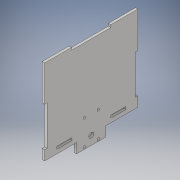
# Autodesk Inventor part: side
Saved by Autodesk Inventor 2019 (Build 230136000, 136)
## iProperties
Created: 2018-09-07
Part Number: side
Material: Generic
Document SubType Name: Modeling
Designer: mspet
Density: 1 g/cm^3
Appearance: Default
Author: mspet
Autodesk Inventor part; units mm, degrees
ref_plane "YZ Plane" through (0, 0, 0) normal (1, 0, 0) x (0, 1, 0)
ref_plane "XZ Plane" through (0, 0, 0) normal (0, 1, 0) x (-1, 0, 0)
ref_plane "XY Plane" through (0, 0, 0) normal (0, 0, 1) x (1, 0, 0)
sketch "Sketch1" plane through (0, 0, 0) normal (1, 0, 0) x (0, 1, 0)
  line L0 (0, 0) -> (97.4344, 0)
  line L1 (97.4344, 0) -> (97.4344, -114.3)
  line L2 (97.4344, -114.3) -> (0, -114.3)
  line L3 (0, -114.3) -> (0, 0)
  dimension "d0" = 114.3
  dimension "d1" = 97.4344
  constraints: 8 end point, 2 parallel, 1 horizontal, 1 perpendicular
  measures "d0" distance of L2.end L0.start
  measures "d1" distance of L1.end L2.end
extrude "Extrusion1" add sketch "Sketch1" along normal blind 3.175
sketch "Sketch2" plane through (3.175, 0, 0) normal (1, 0, 0) x (0, 0, -1)
  circle A0 centre (48.1457, 35.5346) radius 1.4986
  circle A1 centre (66.1543, 35.5346) radius 1.4986
  circle A2 centre (66.1543, 2.54) radius 1.4986
  circle A3 centre (48.1457, 2.54) radius 1.4986
  line L0 (114.3, 0) -> (114.3, 97.4344) projected
  line L1 (0, 0) -> (114.3, 0) projected
  line L2 (0, 0) -> (0, 97.4344) projected
  dimension "d4" = 18.0086
  dimension "d5" = 2.9972
  dimension "d6" = 2.9972
  dimension "d7" = 2.9972
  dimension "d8" = 2.9972
  dimension "d11" = 18.0086
  dimension "d12" = 2.54
  dimension "d28" = 2.54
  dimension "d29" = 32.9946
  dimension "d30" = 32.9946
  dimension "d65" = 48.1457
  constraints: 4 centre point
  measures "d4" distance of A1.centre A0.centre
  measures "d5" diameter of A1
  measures "d6" diameter of A0
  measures "d7" diameter of A3
  measures "d8" diameter of A2
  measures "d11" distance of A2.centre A3.centre
  measures "d12" distance from line of L1 A3.centre
  measures "d28" distance from line of L1 A2.centre
  measures "d29" distance of A2.centre A1.centre
  measures "d30" distance of A3.centre A0.centre
  measures "d65" distance from line of L0 A1.centre
extrude "Extrusion2" cut sketch "Sketch2" against normal blind 3.175
sketch "Sketch3" plane through (3.175, 0, 0) normal (1, 0, 0) x (0, 0, -1)
  circle A0 centre (57.15, 11.5316) radius 3.175
  line L0 (114.3, 0) -> (114.3, 97.4344) projected
  circle A1 centre (66.1543, 2.54) radius 1.4986 projected
  point P0 (0, 0)
  dimension "d15" = 6.35
  dimension "d16" = 57.15
  dimension "d17" = 8.9916
  constraints: 1 centre point
  measures "d15" diameter of A0
  measures "d16" distance from line of L0 A0.centre
  measures "d17" vertical distance of A1.centre A0.centre
extrude "Extrusion3" cut sketch "Sketch3" against normal blind 3.175 contours A0
sketch "Sketch4" plane through (3.175, 0, 0) normal (1, 0, 0) x (0, 0, -1)
  line L0 (0, 97.4344) -> (0, 0) projected
  line L1 (0, 0) -> (114.3, 0) projected
  line L2 (114.3, 0) -> (114.3, 97.4344) projected
  line L3 (31.75, 18.0594) -> (12.7, 18.0594)
  line L4 (12.7, 18.0594) -> (12.7, 21.2344)
  line L5 (12.7, 21.2344) -> (31.75, 21.2344)
  line L6 (31.75, 21.2344) -> (31.75, 18.0594)
  circle A0 centre (57.15, 11.5316) radius 3.175 projected
  line L7 (57.15, 11.5316) -> (57.15, 79.1299) construction
  line L8 (82.55, 18.0594) -> (101.6, 18.0594)
  line L9 (101.6, 18.0594) -> (101.6, 21.2344)
  line L10 (101.6, 21.2344) -> (82.55, 21.2344)
  line L11 (82.55, 21.2344) -> (82.55, 18.0594)
  point P0 (12.7, 0)
  point P1 (31.75, 0)
  point P2 (101.6, 0)
  dimension "d31" = 3.175
  dimension "d33" = 19.05
  dimension "d34" = 12.7
  dimension "d43" = 18.0594
  constraints: 18 end point, 4 symmetric about line, 2 parallel, 1 horizontal, 1 perpendicular, 1 point on line, 1 vertical
  measures "d31" distance of L3.end L4.end
  measures "d33" distance of L4.end L5.end
  measures "d34" distance between parallel lines of L0 L4
  measures "d43" distance between parallel lines of L1 L3
extrude "Extrusion5" cut sketch "Sketch4" against normal blind 3.175 contours L3 L4 L5 L6 | L11 L10 L9 L8
sketch "Sketch5" plane through (3.175, 0, 0) normal (1, 0, 0) x (0, 0, -1)
  line L0 (0, 0) -> (38.1, 0)
  line L1 (38.1, 0) -> (38.1, 12.7)
  line L2 (38.1, 12.7) -> (0, 12.7)
  line L3 (0, 12.7) -> (0, 0)
  line L4 (114.3, 0) -> (0, 0) projected
  line L5 (114.3, 0) -> (76.2, 0)
  line L6 (76.2, 0) -> (76.2, 12.7)
  line L7 (76.2, 12.7) -> (114.3, 12.7)
  line L8 (114.3, 12.7) -> (114.3, 0)
  dimension "d37" = 38.1
  dimension "d38" = 12.7
  dimension "d39" = 38.1
  dimension "d42" = 12.7
  constraints: 16 end point, 4 parallel, 2 horizontal, 2 perpendicular
  measures "d37" distance of L1.end L2.end
  measures "d38" distance of L0.end L1.end
  measures "d39" distance of L6.end L7.end
  measures "d42" distance of L5.end L6.end
extrude "Extrusion6" cut sketch "Sketch5" against normal blind 3.175
sketch "Sketch6" plane through (3.175, 0, 0) normal (1, 0, 0) x (0, 0, -1)
  line L0 (0, 97.4344) -> (0, 12.7) projected
  line L1 (0, 69.85) -> (3.175, 69.85)
  line L2 (3.175, 69.85) -> (3.175, 50.8)
  line L3 (3.175, 50.8) -> (0, 50.8)
  line L4 (0, 50.8) -> (0, 69.85)
  line L5 (0, 12.7) -> (38.1, 12.7) projected
  line L6 (38.1, 0) -> (76.2, 0) projected
  line L7 (57.15, 0) -> (57.15, 76.8026) construction
  line L8 (114.3, 97.4344) -> (114.3, 12.7)
  line L9 (114.3, 69.85) -> (111.125, 69.85)
  line L10 (111.125, 69.85) -> (111.125, 50.8)
  line L11 (111.125, 50.8) -> (114.3, 50.8)
  line L12 (114.3, 50.8) -> (114.3, 69.85)
  point P0 (0, 0)
  dimension "d44" = 38.1
  dimension "d45" = 19.05
  dimension "d46" = 3.175
  constraints: 20 end point, 6 symmetric about line, 2 parallel, 2 point on line, 1 horizontal, 1 midpoint, 1 perpendicular, 1 vertical
  measures "d44" distance between parallel lines of L3 L5
  measures "d45" distance of L1.end L2.end
  measures "d46" distance of L1.start L1.end
extrude "Extrusion7" cut sketch "Sketch6" against normal blind 3.175
sketch "Sketch7" plane through (3.175, 0, 0) normal (1, 0, 0) x (0, 0, -1)
  line L0 (0, 101.4731) -> (-3.175, 101.4731)
  line L1 (-3.175, 101.4731) -> (-3.175, 12.7)
  line L2 (-3.175, 12.7) -> (0, 12.7)
  line L3 (0, 12.7) -> (0, 101.4731)
  line L4 (114.3, 50.8) -> (114.3, 12.7) projected
  line L5 (114.3, 12.7) -> (117.475, 12.7)
  line L6 (117.475, 12.7) -> (117.475, 101.4731)
  line L7 (117.475, 101.4731) -> (114.3, 101.4731)
  line L8 (114.3, 101.4731) -> (114.3, 12.7)
  line L9 (0, 97.4344) -> (0, 69.85) projected
  line L10 (0, 69.85) -> (3.3446, 69.85)
  line L11 (3.3446, 69.85) -> (3.3446, 50.8)
  line L12 (3.3446, 50.8) -> (0, 50.8)
  line L13 (0, 50.8) -> (0, 69.85)
  line L14 (111.125, 69.85) -> (111.125, 50.8) projected
  line L15 (111.125, 69.85) -> (114.3, 69.85)
  line L16 (114.3, 69.85) -> (114.3, 50.8)
  line L17 (114.3, 50.8) -> (111.125, 50.8)
  line L18 (111.125, 50.8) -> (111.125, 69.85)
  line L19 (0, 97.4344) -> (-3.175, 97.4344)
  line L20 (0, 97.4344) -> (114.3, 97.4344) projected
  line L21 (114.3, 97.4344) -> (117.475, 97.4344)
  point P0 (0, 0)
  dimension "d49" = 3.175
  dimension "d50" = 3.175
  dimension "d51" = 0
  constraints: 36 end point, 8 parallel, 6 perpendicular, 4 horizontal, 3 point on line
  measures "d49" distance of L0.start L0.end
  measures "d50" distance of L6.end L7.end
  measures "d51" distance between parallel lines of L9 L3
extrude "Extrusion8" add sketch "Sketch7" against normal blind 3.175
sketch "Sketch8" plane through (3.175, 0, 0) normal (1, 0, 0) x (0, 0, -1)
  line L0 (-3.175, 101.4731) -> (-3.175, 12.7) projected
  line L1 (-3.175, 76.2) -> (0, 76.2)
  line L2 (0, 76.2) -> (0, 25.4)
  line L3 (0, 25.4) -> (-3.175, 25.4)
  line L4 (-3.175, 25.4) -> (-3.175, 76.2)
  line L5 (117.475, 101.4731) -> (117.475, 12.7) projected
  line L6 (117.475, 76.2) -> (114.3, 76.2)
  line L7 (114.3, 76.2) -> (114.3, 25.4)
  line L8 (114.3, 25.4) -> (117.475, 25.4)
  line L9 (117.475, 25.4) -> (117.475, 76.2)
  line L10 (-3.175, 12.7) -> (38.1, 12.7) projected
  point P0 (0, 0)
  dimension "d54" = 3.175
  dimension "d55" = 3.175
  dimension "d56" = 50.8
  dimension "d57" = 50.8
  dimension "d58" = 12.7
  constraints: 16 end point, 4 parallel, 3 point on line, 2 horizontal, 2 perpendicular
  measures "d54" distance of L7.end L8.end
  measures "d55" distance of L1.start L1.end
  measures "d56" distance of L1.end L2.end
  measures "d57" distance of L6.end L7.end
  measures "d58" distance between parallel lines of L10 L3
extrude "Extrusion9" cut sketch "Sketch8" against normal blind 3.175
sketch "Sketch9" plane through (3.175, 0, 0) normal (1, 0, 0) x (0, 0, -1)
  line L0 (-3.175, 76.2) -> (-3.175, 101.4731) projected
  line L1 (-3.175, 97.0871) -> (127.7131, 97.0871)
  line L2 (127.7131, 97.0871) -> (127.7131, 110.1997)
  line L3 (127.7131, 110.1997) -> (-3.175, 110.1997)
  line L4 (-3.175, 110.1997) -> (-3.175, 97.0871)
  point P0 (0, 0)
  constraints: 8 end point, 2 parallel, 1 horizontal, 1 perpendicular, 1 point on line
extrude "Extrusion10" cut sketch "Sketch9" against normal blind 3.175
sketch "Sketch10" plane through (0, 0, 0) normal (-1, 0, 0) x (0, 0, 1)
  line L0 (-117.475, 97.0871) -> (-117.475, 76.2) projected
  line L1 (-117.475, 97.0871) -> (3.175, 97.0871)
  line L2 (3.175, 97.0871) -> (3.175, 122.4871)
  line L3 (3.175, 122.4871) -> (-117.475, 122.4871)
  line L4 (-117.475, 122.4871) -> (-117.475, 97.0871)
  line L5 (3.175, 76.2) -> (3.175, 97.0871) projected
  point P0 (0, 0)
  dimension "d66" = 0
  dimension "d67" = 25.4
  constraints: 8 end point, 2 parallel, 1 horizontal, 1 perpendicular
  measures "d66" distance between parallel lines of L2 L5
  measures "d67" distance of L3.end L0.start
extrude "Extrusion11" add sketch "Sketch10" against normal blind 3.175
sketch "Sketch11" plane through (3.175, 0, 0) normal (1, 0, 0) x (0, 0, -1)
  line L0 (117.475, 122.4871) -> (-3.175, 122.4871) projected
  line L1 (31.75, 122.4871) -> (82.55, 122.4871)
  line L2 (82.55, 122.4871) -> (82.55, 119.3121)
  line L3 (82.55, 119.3121) -> (31.75, 119.3121)
  line L4 (31.75, 119.3121) -> (31.75, 122.4871)
  line L5 (-3.175, 122.4871) -> (-3.175, 76.2) projected
  point P0 (0, 0)
  dimension "d70" = 50.8
  dimension "d71" = 3.175
  dimension "d72" = 34.925
  constraints: 8 end point, 2 parallel, 1 horizontal, 1 perpendicular, 1 point on line
  measures "d70" distance of L2.end L3.end
  measures "d71" distance of L1.end L2.end
  measures "d72" distance between parallel lines of L5 L4
extrude "Extrusion12" cut sketch "Sketch11" against normal blind 3.175
body "Solid1"
